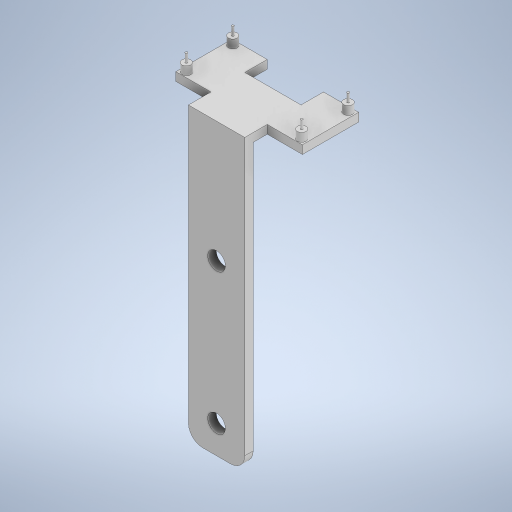
# Autodesk Inventor part: sonic_sensor_holder
Saved by Autodesk Inventor 2024.3 (Build 283343000, 343)
## iProperties
Created: 2025-10-17
Part Number: sonic_sensor_holder
Material: 일반
Document SubType Name: Modeling
Designer: joung
Density: 1 g/cm^3
Appearance: 기본값
Author: joung
Autodesk Inventor part; units mm, degrees
ref_plane "YZ Plane" through (0, 0, 0) normal (1, 0, 0) x (0, 1, 0)
ref_plane "XZ Plane" through (0, 0, 0) normal (0, 1, 0) x (-1, 0, 0)
ref_plane "XY Plane" through (0, 0, 0) normal (0, 0, 1) x (1, 0, 0)
sketch "스케치1" plane through (0, 0, 0) normal (0, 1, 0) x (-1, 0, 0)
  line L0 (20.5, 10) -> (-20.5, 10)
  line L1 (-22.5, 8) -> (-22.5, -8)
  line L2 (-20.5, -10) -> (20.5, -10)
  line L3 (22.5, -8) -> (22.5, 8)
  line L4 (22.5, 10) -> (-22.5, -10) construction
  line L5 (-22.5, 10) -> (22.5, -10) construction
  line L6 (20.5, 8.25) -> (-20.5, 8.25)
  line L7 (-20.5, 8.25) -> (-20.5, -8.25)
  line L8 (-20.5, -8.25) -> (20.5, -8.25)
  line L9 (20.5, -8.25) -> (20.5, 8.25)
  line L10 (20.5, 8.25) -> (-20.5, -8.25) construction
  line L11 (-20.5, 8.25) -> (20.5, -8.25) construction
  circle A0 centre (20.5, -8.25) radius 1.1
  circle A1 centre (-20.5, -8.25) radius 1.1
  circle A2 centre (-20.5, 8.25) radius 1.1
  circle A3 centre (20.5, 8.25) radius 1.1
  arc A4 (20.5, -10) -> (22.5, -8) centre (20.5, -8) ccw
  arc A5 (22.5, 8) -> (20.5, 10) centre (20.5, 8) ccw
  arc A6 (-20.5, 10) -> (-22.5, 8) centre (-20.5, 8) ccw
  arc A7 (-22.5, -8) -> (-20.5, -10) centre (-20.5, -8) ccw
  line L12 (-22.5, 10) -> (22.5, 10)
  line L13 (22.5, 10) -> (22.5, -10)
  line L14 (22.5, -10) -> (-22.5, -10)
  line L15 (-22.5, -10) -> (-22.5, 10)
  line L16 (-22.5, 10) -> (22.5, -10) construction
  line L17 (22.5, 10) -> (-22.5, -10) construction
  point P0 (0, 0)
  dimension "d0" = 45
  dimension "d1" = 20
  dimension "d2" = 41
  dimension "d3" = 16.5
  dimension "d4" = 2.2
  dimension "d5" = 2.2
  dimension "d6" = 2.2
  dimension "d7" = 2.2
  dimension "d8" = 2
  constraints: 36 end point, 8 centre point, 8 point on circle, 8 point on line, 8 tangent, 6 midpoint, 6 parallel, 4 coincident, 3 equal radius, 3 horizontal, 3 perpendicular
  measures "d0" distance of L5.end L4.end
  measures "d1" distance of L4.end L5.start
  measures "d2" distance of L8.end L7.end
  measures "d3" distance of L7.end L6.end
  measures "d4" diameter of A0
  measures "d5" diameter of A1
  measures "d6" diameter of A2
  measures "d7" diameter of A3
  measures "d8" radius of A4
extrude "돌출1" add sketch "스케치1" along normal blind 3 contours A5 L3 A4 L2 A7 L1 A6 L0 | L12 L13 A5 | A6 L15 L12 | L13 L14 A4 | A7 L14 L15 | L6 A3 L9 A0 L8 A1 L7 A2
sketch "스케치6" plane through (-22.5, 0, 10) normal (0, 0, 1) x (1, 0, 0)
  line L0 (45, 3) -> (0, 3) projected
  line L1 (12.5, 0) -> (32.5, 0)
  line L2 (32.5, 0) -> (32.5, 3)
  line L3 (32.5, 3) -> (12.5, 3)
  line L4 (12.5, 3) -> (12.5, 0)
  line L5 (12.5, 0) -> (32.5, 3) construction
  line L6 (32.5, 0) -> (12.5, 3) construction
  point P0 (22.5, 0)
  point P1 (22.5, 1.5)
  dimension "d23" = 20
  constraints: 12 end point, 2 midpoint, 2 parallel, 1 horizontal, 1 perpendicular, 1 point on line
  measures "d23" distance of L3.end L2.end
extrude "돌출5" add sketch "스케치6" along normal blind 8
sketch "스케치7" plane through (0, 0, 0) normal (0, -1, 0) x (1, 0, 0)
  line L0 (-10, 18) -> (10, 18) projected
  line L1 (-10, 10) -> (-10, 18) projected
  line L2 (10, 18) -> (-10, 18)
  line L3 (-10, 18) -> (-10, 15)
  line L4 (-10, 15) -> (10, 15)
  line L5 (10, 15) -> (10, 18)
  point P0 (0, 0)
  dimension "d26" = 3
  constraints: 8 end point, 2 parallel, 1 horizontal, 1 perpendicular, 1 point on line
  measures "d26" distance of L3.end L2.end
extrude "돌출6" add sketch "스케치7" along normal blind 100
sketch "스케치8" plane through (10, 0, 15) normal (0, 0, -1) x (-1, 0, 0)
  line L0 (20, -100) -> (0, -100) projected
  line L1 (10, -100) -> (10, -90)
  line L2 (10, -90) -> (10, -40)
  circle A0 centre (10, -40) radius 3.15
  circle A1 centre (10, -90) radius 3.15
  point P0 (10, 0)
  dimension "d29" = 10
  dimension "d30" = 50
  dimension "d31" = 6.3
  dimension "d32" = 6.3
  constraints: 4 end point, 2 centre point, 2 coincident, 1 midpoint, 1 point on line, 1 vertical
  measures "d29" distance of L1.start L1.end
  measures "d30" distance of L1.end L2.end
  measures "d31" diameter of A0
  measures "d32" diameter of A1
extrude "돌출7" cut sketch "스케치8" against normal blind 100
sketch "스케치9" plane through (0, 3, 0) normal (0, 1, 0) x (1, 0, 0)
  circle A0 centre (-20.5, 8.25) radius 1.1 projected
  circle A1 centre (-20.5, 8.25) radius 1.1
  circle A2 centre (-20.5, 8.25) radius 1.6
  line L0 (22.5, 10) -> (-22.5, 10) projected
  line L1 (0, 10) -> (0, -18)
  line L2 (10, -18) -> (-10, -18) projected
  line L3 (-22.5, 10) -> (-22.5, -10) projected
  line L4 (-22.5, 0) -> (22.5, 0)
  line L5 (22.5, -10) -> (22.5, 10) projected
  circle A3 centre (20.5, 8.25) radius 1.1
  circle A4 centre (20.5, 8.25) radius 1.1
  circle A5 centre (20.5, 8.25) radius 1.6
  circle A6 centre (-20.5, -8.25) radius 1.1
  circle A7 centre (-20.5, -8.25) radius 1.1
  circle A8 centre (-20.5, -8.25) radius 1.6
  line L6 (22.5, -10) -> (-22.5, -10)
  circle A9 centre (20.5, -8.25) radius 1.1
  circle A10 centre (20.5, -8.25) radius 1.1
  circle A11 centre (20.5, -8.25) radius 1.6
  point P0 (0, 0)
  point P1 (0, -10)
  dimension "d35" = 0.5
  constraints: 11 centre point, 7 symmetric about line, 6 end point, 4 coincident, 4 midpoint, 9 other
  measures "d35" radial gap between concentric circles of A0 A2
extrude "돌출8" add sketch "스케치9" along normal blind 3 contours A2 | A5 | A8 | A11
sketch "스케치10" plane through (0, 3, 0) normal (0, 1, 0) x (1, 0, 0)
  line L0 (22.5, 10) -> (-22.5, 10) projected
  line L1 (0, 10) -> (-10, 10)
  line L2 (0, 10) -> (10, 10) construction
  line L3 (-10, 10) -> (10, 10)
  line L4 (10, 10) -> (10, 2)
  line L5 (10, 2) -> (-10, 2)
  line L6 (-10, 2) -> (-10, 10)
  point P0 (0, 0)
  dimension "d38" = 10
  dimension "d39" = 180
  dimension "d40" = 20
  dimension "d41" = 8
  constraints: 12 end point, 2 collinear, 2 horizontal, 2 parallel, 1 midpoint, 1 perpendicular
  measures "d38" distance of L1.start L1.end
  measures "d39" angle of L1 L2
  measures "d40" distance of L4.end L5.end
  measures "d41" distance of L3.end L4.end
extrude "돌출9" cut sketch "스케치10" against normal blind 3
fillet "모깎기1" radius 5 2 edges at (-10, -100, 16.5) (10, -100, 16.5)
sketch "스케치11" plane through (-20.5, 6, -8.25) normal (0, 1, 0) x (1, 0, 0)
  circle A0 centre (0, 0) radius 1.1 projected
  circle A1 centre (0, 0) radius 1.1
  circle A2 centre (0, -16.5) radius 1.1 projected
  circle A3 centre (0, -16.5) radius 1.1
  circle A4 centre (41, 0) radius 1.1 projected
  circle A5 centre (41, 0) radius 1.1
  circle A6 centre (41, -16.5) radius 1.1 projected
  circle A7 centre (41, -16.5) radius 1.1
  point P0 (20.5, -8.25)
  constraints: 4 centre point, 4 coincident
extrude "돌출10" add sketch "스케치11" against normal up to surface (6 mm away)
sketch "스케치12" plane through (20.5, 6, -8.25) normal (0, 1, 0) x (1, 0, 0)
  circle A0 centre (-41, 0) radius 1.6 projected
  circle A1 centre (-41, 0) radius 0.4
  circle A2 centre (-41, -16.5) radius 1.6 projected
  circle A3 centre (-41, -16.5) radius 0.4
  circle A4 centre (0, 0) radius 1.6 projected
  circle A5 centre (0, 0) radius 0.4
  circle A6 centre (0, -16.5) radius 1.6 projected
  circle A7 centre (0, -16.5) radius 0.4
  point P0 (-20.5, -8.25)
  dimension "d47" = 0.8
  dimension "d48" = 0.8
  dimension "d49" = 0.8
  dimension "d50" = 0.8
  constraints: 4 centre point, 4 coincident
  measures "d47" diameter of A1
  measures "d48" diameter of A3
  measures "d49" diameter of A5
  measures "d50" diameter of A7
extrude "돌출11" add sketch "스케치12" along normal blind 3 contours A1 | A3 | A5 | A7
